Autodesk Inventor part; units mm, degrees
(part 2 of 2)
sketch "Sketch21" plane through (0, 18, 0) normal (0, 1, 0) x (1, 0, 0)
  line L0 (-120.65, 106.3625) -> (-120.65, 90.4875) projected
  line L1 (-120.65, 106.3625) -> (-120.65, 92.3625)
  line L2 (-120.65, 106.3625) -> (-120.65, 92.3625)
  line L3 (-147.6375, 92.3625) -> (-147.6375, 87.3625)
  line L4 (-147.6375, 87.3625) -> (-147.6375, 73.3625)
  line L5 (-147.6375, 73.3625) -> (-147.6375, 68.3625)
  line L6 (-147.6375, 68.3625) -> (-147.6375, 54.3625)
  line L7 (-147.6375, 54.3625) -> (-147.6375, 49.3625)
  line L8 (-147.6375, 49.3625) -> (-147.6375, 35.3625)
  line L9 (-147.6375, 35.3625) -> (-147.6375, 30.3625)
  line L10 (-147.6375, 30.3625) -> (-147.6375, 16.3625)
  line L11 (-147.6375, 16.3625) -> (-147.6375, 11.3625)
  line L12 (-147.6375, 11.3625) -> (-147.6375, -2.6375)
  line L13 (-147.6375, -2.6375) -> (-147.6375, -7.6375)
  line L14 (-147.6375, -7.6375) -> (-147.6375, -21.6375)
  line L15 (-147.6375, -21.6375) -> (-147.6375, -26.6375)
  line L16 (-147.6375, -26.6375) -> (-147.6375, -40.6375)
  line L17 (-147.6375, -40.6375) -> (-147.6375, -45.6375)
  line L18 (-147.6375, -45.6375) -> (-147.6375, -59.6375)
  line L19 (-147.6375, -59.6375) -> (-147.6375, -64.6375)
  line L20 (-147.6375, -64.6375) -> (-147.6375, -78.6375)
  line L21 (-147.6375, -78.6375) -> (-147.6375, -83.6375)
  line L22 (-147.6375, -83.6375) -> (-147.6375, -97.6375)
  line L23 (-147.6375, -97.6375) -> (-147.6375, -102.6375)
  line L24 (-147.6375, -102.6375) -> (-147.6375, -116.6375)
  line L25 (-147.6375, -116.6375) -> (-147.6375, -121.6375)
  line L26 (-147.6375, -121.6375) -> (-147.6375, -135.6375)
  line L27 (-117.475, -138.223) -> (-117.475, -117.223) projected
  line L28 (-29.225, 139.5812) -> (-148.575, 139.5812) projected
  line L29 (-120.65, 106.3625) -> (-120.65, 92.3625)
  line L30 (-120.65, 92.3625) -> (-134.65, 92.3625)
  line L31 (-134.65, 92.3625) -> (-134.65, 106.3625)
  line L32 (-134.65, 106.3625) -> (-120.65, 106.3625)
  line L33 (-120.65, 87.3625) -> (-120.65, 73.3625)
  line L34 (-120.65, 73.3625) -> (-134.65, 73.3625)
  line L35 (-134.65, 73.3625) -> (-134.65, 87.3625)
  line L36 (-134.65, 87.3625) -> (-120.65, 87.3625)
  line L37 (-134.65, 73.3625) -> (-120.65, 73.3625)
  line L38 (-120.65, 68.3625) -> (-120.65, 54.3625)
  line L39 (-120.65, 54.3625) -> (-134.65, 54.3625)
  line L40 (-134.65, 54.3625) -> (-134.65, 68.3625)
  line L41 (-134.65, 68.3625) -> (-120.65, 68.3625)
  line L42 (-134.65, 54.3625) -> (-120.65, 54.3625)
  line L43 (-120.65, 49.75) -> (-120.65, 35.75)
  line L44 (-120.65, 49.75) -> (-120.65, 35.75)
  line L45 (-120.65, 35.75) -> (-134.65, 35.75)
  line L46 (-134.65, 35.75) -> (-134.65, 49.75)
  line L47 (-120.65, 49.75) -> (-120.65, 35.75)
  line L48 (-134.65, 49.75) -> (-120.65, 49.75)
  line L49 (-120.65, 16.75) -> (-134.65, 16.75)
  line L50 (-134.65, 16.75) -> (-134.65, 30.75)
  line L51 (-120.65, 30.75) -> (-120.65, 16.75)
  line L52 (-134.65, 30.75) -> (-120.65, 30.75)
  line L53 (-134.65, 16.75) -> (-120.65, 16.75)
  line L54 (-120.65, -2.25) -> (-134.65, -2.25)
  line L55 (-134.65, -2.25) -> (-134.65, 11.75)
  line L56 (-120.65, 11.75) -> (-120.65, -2.25)
  line L57 (-134.65, 11.75) -> (-120.65, 11.75)
  line L58 (-134.65, -2.25) -> (-120.65, -2.25)
  line L59 (-120.65, -7.25) -> (-120.65, -21.25)
  line L60 (-120.65, -7.25) -> (-120.65, -21.25)
  line L61 (-120.65, -21.25) -> (-134.65, -21.25)
  line L62 (-134.65, -21.25) -> (-134.65, -7.25)
  line L63 (-120.65, -7.25) -> (-120.65, -21.25)
  line L64 (-134.65, -7.25) -> (-120.65, -7.25)
  line L65 (-120.65, -40.25) -> (-134.65, -40.25)
  line L66 (-134.65, -40.25) -> (-134.65, -26.25)
  line L67 (-120.65, -26.25) -> (-120.65, -40.25)
  line L68 (-134.65, -26.25) -> (-120.65, -26.25)
  line L69 (-134.65, -40.25) -> (-120.65, -40.25)
  line L70 (-120.65, -59.25) -> (-134.65, -59.25)
  line L71 (-134.65, -59.25) -> (-134.65, -45.25)
  line L72 (-120.65, -45.25) -> (-120.65, -59.25)
  line L73 (-134.65, -45.25) -> (-120.65, -45.25)
  line L74 (-134.65, -59.25) -> (-120.65, -59.25)
  line L75 (-120.65, -64.8355) -> (-120.65, -78.8355)
  line L76 (-120.65, -64.8355) -> (-120.65, -78.8355)
  line L77 (-120.65, -78.8355) -> (-134.65, -78.8355)
  line L78 (-134.65, -78.8355) -> (-134.65, -64.8355)
  line L79 (-120.65, -64.8355) -> (-120.65, -78.8355)
  line L80 (-134.65, -64.8355) -> (-120.65, -64.8355)
  line L81 (-120.65, -97.8355) -> (-134.65, -97.8355)
  line L82 (-134.65, -97.8355) -> (-134.65, -83.8355)
  line L83 (-120.65, -83.8355) -> (-120.65, -97.8355)
  line L84 (-134.65, -83.8355) -> (-120.65, -83.8355)
  line L85 (-134.65, -97.8355) -> (-120.65, -97.8355)
  line L86 (-134.65, -116.8355) -> (-134.65, -102.8355)
  line L87 (-120.65, -102.8355) -> (-120.65, -116.8355)
  line L88 (-120.65, -85.8355) -> (-120.65, -99.8355)
  line L89 (-120.65, -85.8355) -> (-120.65, -99.8355)
  line L90 (-134.65, -99.8355) -> (-134.65, -85.8355)
  line L91 (-120.65, -85.8355) -> (-120.65, -99.8355)
  line L92 (-120.65, -118.8355) -> (-134.65, -118.8355)
  line L93 (-134.65, -118.8355) -> (-134.65, -104.8355)
  line L94 (-120.65, -104.8355) -> (-120.65, -118.8355)
  line L95 (-134.65, -104.8355) -> (-120.65, -104.8355)
  line L96 (-134.65, -118.8355) -> (-120.65, -118.8355)
  line L97 (-120.65, -137.8355) -> (-134.65, -137.8355)
  line L98 (-134.65, -137.8355) -> (-134.65, -123.8355)
  line L99 (-120.65, -123.8355) -> (-120.65, -137.8355)
  line L100 (-134.65, -123.8355) -> (-120.65, -123.8355)
  line L101 (-134.65, -137.8355) -> (-120.65, -137.8355)
  point P0 (0, 0)
  point P1 (-120.65, 49.0875)
  point P2 (-120.65, -7.9125)
  point P3 (-120.65, -65.498)
  point P4 (-120.65, -86.498)
  dimension "d213" = 5
  dimension "d214" = 14
  dimension "d215" = 5
  dimension "d216" = 14
  dimension "d217" = 5
  dimension "d218" = 14
  dimension "d219" = 5
  dimension "d220" = 14
  dimension "d221" = 5
  dimension "d222" = 14
  dimension "d223" = 5
  dimension "d224" = 14
  dimension "d225" = 5
  dimension "d226" = 14
  dimension "d227" = 5
  dimension "d228" = 14
  dimension "d229" = 5
  dimension "d230" = 14
  dimension "d231" = 5
  dimension "d232" = 14
  dimension "d233" = 5
  dimension "d234" = 14
  dimension "d235" = 5
  dimension "d236" = 14
  dimension "d239" = 14
  dimension "d255" = 14
  dimension "d256" = 14
  dimension "d257" = 14
  constraints: 198 end point, 26 perpendicular, 23 point on line, 1 vertical
  measures "d213" distance of L3.start L3.end
  measures "d214" distance of L3.end L4.end
  measures "d215" distance of L4.end L5.end
  measures "d216" distance of L5.end L6.end
  measures "d217" distance of L6.end L7.end
  measures "d218" distance of L7.end L8.end
  measures "d219" distance of L8.end L9.end
  measures "d220" distance of L9.end L10.end
  measures "d221" distance of L10.end L11.end
  measures "d222" distance of L11.end L12.end
  measures "d223" distance of L12.end L13.end
  measures "d224" distance of L13.end L14.end
  measures "d225" distance of L14.end L15.end
  measures "d226" distance of L15.end L16.end
  measures "d227" distance of L16.end L17.end
  measures "d228" distance of L17.end L18.end
  measures "d229" distance of L18.end L19.end
  measures "d230" distance of L19.end L20.end
  measures "d231" distance of L20.end L21.end
  measures "d232" distance of L21.end L22.end
  measures "d233" distance of L22.end L23.end
  measures "d234" distance of L23.end L24.end
  measures "d235" distance of L24.end L25.end
  measures "d236" distance of L25.end L26.end
  measures "d239" distance of L29.start L30.start
  measures "d255" distance of L48.end L45.start
  measures "d256" distance of L64.end L61.start
  measures "d257" distance of L80.end L77.start
extrude "Extrusion15" add sketch "Sketch21" along normal blind 2
extrude "Extrusion16" add sketch "Sketch2" along normal blind 0.1 contours L26 L23 A5 L25 L43 A9 L42 A6 L41 A7 L36 L19
thicken "Thicken1" operation add thickness 1 both sides no extend neighbours yes toward (0, 1, 0) faces at (-131.2333, 13, 79.9042)
extrude "Extrusion17" add sketch "Sketch18" along normal blind 1
extrude "Extrusion18" add sketch "Sketch2" along normal blind 18 contours L26 L23 A5 L25 L43 A9 L42 A6 L41 A7 L36 L19
sketch "Sketch22" plane through (0, 20, 0) normal (0, 1, 0) x (1, 0, 0)
  point P0 (0, 0)
sketch "Sketch23" plane through (0, 18, 0) normal (0, 1, 0) x (1, 0, 0)
  line L0 (-65.0875, -55.7625) -> (-80.0875, -55.7625) projected
  line L1 (-80.0875, -60.7625) -> (-80.0875, -74.7625)
  line L2 (-80.0875, -79.7625) -> (-80.0875, -93.7625)
  line L3 (-80.0875, -98.7625) -> (-65.0875, -98.7625)
  line L4 (-65.0875, -79.7625) -> (-80.0875, -79.7625)
  line L5 (-80.0875, -74.7625) -> (-65.0875, -74.7625)
  line L6 (-65.0875, -74.7625) -> (-65.0875, -60.7625)
  line L7 (-65.0875, -60.7625) -> (-80.0875, -60.7625)
  line L8 (-80.0875, -93.7625) -> (-65.0875, -93.7625)
  line L9 (-65.0875, -93.7625) -> (-65.0875, -79.7625)
  line L10 (-80.0875, -98.7625) -> (-80.0875, -138.1125)
  line L11 (-80.0875, -138.1125) -> (-65.0875, -138.1125)
  line L12 (-65.0875, -138.1125) -> (-65.0875, -98.7625)
  line L13 (-80.0875, -98.7625) -> (-80.0875, -112.7625)
  line L14 (-80.0875, -112.7625) -> (-65.0875, -112.7625)
  line L15 (-65.0875, -118.4375) -> (-80.0875, -118.4375)
  line L16 (-80.0875, -118.4375) -> (-80.0875, -112.7625)
  point P0 (0, 0)
  dimension "d269" = 5
  dimension "d270" = 14
  dimension "d271" = 5
  dimension "d272" = 14
  dimension "d273" = 5
  dimension "d274" = 14
  constraints: 32 end point, 7 perpendicular, 4 point on line, 2 midpoint, 1 collinear, 1 horizontal, 1 parallel, 1 vertical
  measures "d269" distance of L0.end L1.start
  measures "d270" distance of L1.start L1.end
  measures "d271" distance of L1.end L2.start
  measures "d272" distance of L2.start L2.end
  measures "d273" distance of L2.end L3.start
  measures "d274" distance of L3.start L13.end
extrude "Extrusion19" add sketch "Sketch23" along normal blind 2 contours L7 L6 L5 L1 | L4 L9 L8 L2 | L3 L12 L14 L10 | L15 L12 L11 L10
sketch "Sketch24" plane through (0, 18, 0) normal (0, 1, 0) x (1, 0, 0)
  line L0 (-80.0875, -118.4375) -> (-65.0875, -118.4375) projected
  line L1 (-65.0875, -112.7125) -> (-65.0875, -118.4375)
  line L2 (-65.0875, -118.4375) -> (-80.0875, -118.4375)
  line L3 (-80.0875, -112.7625) -> (-80.0875, -98.7625) projected
  line L4 (-80.0875, -118.4375) -> (-80.0875, -112.7625)
  line L5 (-65.0875, -98.7625) -> (-65.0875, -112.7625) projected
  line L6 (-80.0875, -112.7625) -> (-65.0875, -112.7625)
  line L7 (-65.0875, -112.7625) -> (-65.0875, -118.4375)
  point P0 (0, 0)
  constraints: 10 end point, 3 perpendicular, 1 collinear, 1 vertical
extrude "Extrusion20" add sketch "Sketch24" along normal blind 1.5
body "Solid1"
body "Srf1"
body "Srf2"
